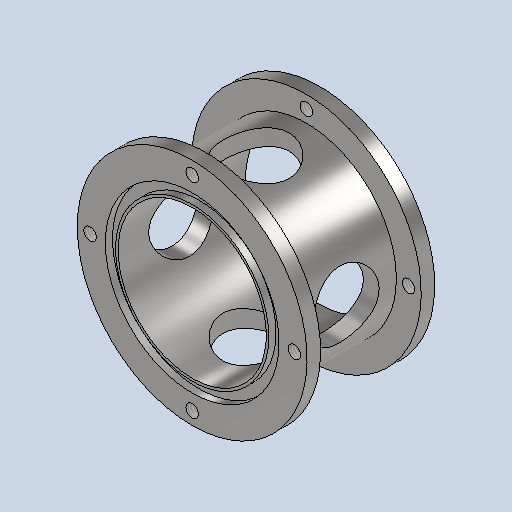
# Autodesk Inventor part: pld_vessel
Saved by Autodesk Inventor 2026 (Build 300175050, 175E)
## iProperties
Created: 2025-11-13
Part Number: pld_vessel
Material: Stainless Steel
Document SubType Name: Modeling
Designer: kuzmin
Density: 8 g/cm^3
Appearance: Semi-Polished
Author: kuzmin
Autodesk Inventor part; units mm, degrees
ref_plane "YZ Plane" through (0, 0, 0) normal (1, 0, 0) x (0, 1, 0)
ref_plane "XZ Plane" through (0, 0, 0) normal (0, 1, 0) x (-1, 0, 0)
ref_plane "XY Plane" through (0, 0, 0) normal (0, 0, 1) x (1, 0, 0)
sketch "Sketch1" plane through (0, 0, 0) normal (1, 0, 0) x (0, 1, 0)
  line L0 (0, 25) -> (0, -25)
  line L1 (-29, 25) -> (-45, 25)
  line L2 (-45, 25) -> (-45, 19.7)
  line L3 (-45, 19.7) -> (-35.25, 19.7)
  line L4 (-35.25, 19.7) -> (-35.25, -19.7)
  line L5 (-35.25, -19.7) -> (-45, -19.7)
  line L6 (-45, -19.7) -> (-45, -25)
  line L7 (-45, -25) -> (-29, -25)
  line L8 (-29, -25) -> (-29, 25)
  point P0 (0, 0)
  point P1 (0, 0)
  point P2 (-29, 0)
  dimension "d0" = 5.3
  dimension "d1" = 50
  dimension "d2" = 90
  dimension "d3" = 70.5
  dimension "d4" = 58
  constraints: 18 end point, 6 perpendicular, 2 horizontal alignment, 2 midpoint, 2 vertical, 1 coincident, 1 collinear, 1 horizontal, 1 vertical alignment
  measures "d0" distance of L1.end L2.end
  measures "d1" distance of L7.end L1.start
  measures "d2" diameter of L2 L0
  measures "d3" diameter of L4 L0
  measures "d4" diameter of L8 L0
revolve "Revolution1" add sketch "Sketch1" angle 360 about axis through (0, 0, 25) along (0, 0, -1)
sketch "Sketch2" plane through (0, 0, 25) normal (0, 0, 1) x (1, 0, 0)
  circle A0 centre (0, 0) radius 30
  circle A1 centre (0, 0) radius 34
  dimension "d6" = 60
  dimension "d7" = 68
  constraints: 2 centre point, 2 coincident
  measures "d6" diameter of A0
  measures "d7" diameter of A1
extrude "Extrusion1" cut sketch "Sketch2" against normal blind 2.8
mirror "Mirror1" about plane through (0, 0, 0) normal (0, 0, 1) of "Extrusion1"
sketch "Sketch3" plane through (0, 0, 25) normal (0, 0, 1) x (1, 0, 0)
  circle A0 centre (0, 0) radius 40 construction
  point P0 (0, 40)
  dimension "d10" = 80
  constraints: 1 coincident, 1 vertical alignment, 2 other
hole "Hole1" at (0, 40, 25) direction (0, 0, -1) diameter 4.917 end through all thread size "M6x1" class "6H" standard "ANSI Metric M Profile"
pattern_circular "Circular Pattern1" count 4 over 360 about axis through (0, 0, 22.35) along (0, 0, -1) of "Hole1"
sketch "Sketch4" plane through (0, 0, 0) normal (1, 0, 0) x (0, 1, 0)
  circle A0 centre (0, 0) radius 13
  dimension "d21" = 26
  constraints: 1 centre point, 1 coincident
  measures "d21" diameter of A0
extrude "Extrusion2" add sketch "Sketch4" along normal mid plane 100 separate body
pattern_circular "Circular Pattern2" count 2 over 90 about axis through (0, 0, -10) along (0, 0, 1) of "Extrusion2" bodies 2
combine bodies "Combine1" operation type subtract main body 1 bodies to subtract 2
body "Solid1"
